Autodesk Inventor part; units mm, degrees
(part 4 of 5)
  arc A370 (116.0375, 307.325) -> (116.5375, 307.825) centre (116.0375, 307.825) ccw
  arc A371 (116.5375, 320.825) -> (116.0375, 321.325) centre (116.0375, 320.825) ccw
  line L372 (102.5375, 326.875) -> (102.5375, 339.875)
  line L373 (116.5375, 326.875) -> (116.5375, 339.875)
  line L374 (103.0375, 326.375) -> (116.0375, 326.375)
  line L375 (103.0375, 340.375) -> (116.0375, 340.375)
  arc A372 (102.5375, 326.875) -> (103.0375, 326.375) centre (103.0375, 326.875) ccw
  arc A373 (103.0375, 340.375) -> (102.5375, 339.875) centre (103.0375, 339.875) ccw
  arc A374 (116.0375, 326.375) -> (116.5375, 326.875) centre (116.0375, 326.875) ccw
  arc A375 (116.5375, 339.875) -> (116.0375, 340.375) centre (116.0375, 339.875) ccw
  line L376 (119.0625, -4.7625) -> (119.0625, 342.9)
  line L377 (0, -4.7625) -> (0, 342.9)
  line L378 (119.0625, -4.7625) -> (0, -4.7625)
  line L379 (119.0625, 342.9) -> (0, 342.9)
  point P0 (60.5977, 160.7988)
sketch "Sketch1" plane through (0, 0, 0) normal (0, 1, 0) x (-1, 0, 0)
  line L0 (0, 0) -> (144.19, 0)
  line L1 (144.19, 0) -> (144.19, -379.14)
  line L2 (144.19, -379.14) -> (0, -379.14)
  line L3 (0, -379.14) -> (0, 0)
  dimension "d0" = 144.19
  dimension "d1" = 379.14
  constraints: 8 end point, 2 parallel, 1 horizontal, 1 perpendicular
  measures "d0" distance of L1.end L2.end
  measures "d1" distance of L0.end L1.end
extrude "Extrusion1" add sketch "Sketch1" along normal blind 2
sketch "Sketch5" plane through (0, 2, 0) normal (0, 1, 0) x (1, 0, 0)
  line L0 (-144.19, 379.14) -> (-144.19, 0) projected
  line L1 (0, 379.14) -> (-144.19, 379.14) projected
  line L2 (0, 0) -> (0, 379.14) projected
  line L3 (-144.19, 0) -> (0, 0) projected
  line L4 (-128.9335, 19.693) -> (-128.9335, 32.693)
  line L5 (-114.9335, 19.693) -> (-114.9335, 32.693)
  line L6 (-128.4335, 19.193) -> (-115.4335, 19.193)
  line L7 (-128.4335, 33.193) -> (-115.4335, 33.193)
  arc A0 (-128.9335, 19.693) -> (-128.4335, 19.193) centre (-128.4335, 19.693) ccw
  arc A1 (-128.4335, 33.193) -> (-128.9335, 32.693) centre (-128.4335, 32.693) ccw
  arc A2 (-115.4335, 19.193) -> (-114.9335, 19.693) centre (-115.4335, 19.693) ccw
  arc A3 (-114.9335, 32.693) -> (-115.4335, 33.193) centre (-115.4335, 32.693) ccw
  line L8 (-128.9335, 57.793) -> (-128.9335, 70.793)
  line L9 (-114.9335, 57.793) -> (-114.9335, 70.793)
  line L10 (-128.4335, 57.293) -> (-115.4335, 57.293)
  line L11 (-128.4335, 71.293) -> (-115.4335, 71.293)
  arc A4 (-128.9335, 57.793) -> (-128.4335, 57.293) centre (-128.4335, 57.793) ccw
  arc A5 (-128.4335, 71.293) -> (-128.9335, 70.793) centre (-128.4335, 70.793) ccw
  arc A6 (-115.4335, 57.293) -> (-114.9335, 57.793) centre (-115.4335, 57.793) ccw
  arc A7 (-114.9335, 70.793) -> (-115.4335, 71.293) centre (-115.4335, 70.793) ccw
  line L12 (-128.9335, 76.843) -> (-128.9335, 89.843)
  line L13 (-114.9335, 76.843) -> (-114.9335, 89.843)
  line L14 (-128.4335, 76.343) -> (-115.4335, 76.343)
  line L15 (-128.4335, 90.343) -> (-115.4335, 90.343)
  arc A8 (-128.9335, 76.843) -> (-128.4335, 76.343) centre (-128.4335, 76.843) ccw
  arc A9 (-128.4335, 90.343) -> (-128.9335, 89.843) centre (-128.4335, 89.843) ccw
  arc A10 (-115.4335, 76.343) -> (-114.9335, 76.843) centre (-115.4335, 76.843) ccw
  arc A11 (-114.9335, 89.843) -> (-115.4335, 90.343) centre (-115.4335, 89.843) ccw
  line L16 (-128.9335, 95.893) -> (-128.9335, 108.893)
  line L17 (-114.9335, 95.893) -> (-114.9335, 108.893)
  line L18 (-128.4335, 95.393) -> (-115.4335, 95.393)
  line L19 (-128.4335, 109.393) -> (-115.4335, 109.393)
  arc A12 (-128.9335, 95.893) -> (-128.4335, 95.393) centre (-128.4335, 95.893) ccw
  arc A13 (-128.4335, 109.393) -> (-128.9335, 108.893) centre (-128.4335, 108.893) ccw
  arc A14 (-115.4335, 95.393) -> (-114.9335, 95.893) centre (-115.4335, 95.893) ccw
  arc A15 (-114.9335, 108.893) -> (-115.4335, 109.393) centre (-115.4335, 108.893) ccw
  line L20 (-128.9335, 114.943) -> (-128.9335, 127.943)
  line L21 (-114.9335, 114.943) -> (-114.9335, 127.943)
  line L22 (-128.4335, 114.443) -> (-115.4335, 114.443)
  line L23 (-128.4335, 128.443) -> (-115.4335, 128.443)
  arc A16 (-128.9335, 114.943) -> (-128.4335, 114.443) centre (-128.4335, 114.943) ccw
  arc A17 (-128.4335, 128.443) -> (-128.9335, 127.943) centre (-128.4335, 127.943) ccw
  arc A18 (-115.4335, 114.443) -> (-114.9335, 114.943) centre (-115.4335, 114.943) ccw
  arc A19 (-114.9335, 127.943) -> (-115.4335, 128.443) centre (-115.4335, 127.943) ccw
  line L24 (-128.9335, 143.518) -> (-128.9335, 156.518)
  line L25 (-114.9335, 143.518) -> (-114.9335, 156.518)
  line L26 (-128.4335, 143.018) -> (-115.4335, 143.018)
  line L27 (-128.4335, 157.018) -> (-115.4335, 157.018)
  arc A20 (-128.9335, 143.518) -> (-128.4335, 143.018) centre (-128.4335, 143.518) ccw
  arc A21 (-128.4335, 157.018) -> (-128.9335, 156.518) centre (-128.4335, 156.518) ccw
  arc A22 (-115.4335, 143.018) -> (-114.9335, 143.518) centre (-115.4335, 143.518) ccw
  arc A23 (-114.9335, 156.518) -> (-115.4335, 157.018) centre (-115.4335, 156.518) ccw
  line L28 (-128.9335, 162.568) -> (-128.9335, 175.568)
  line L29 (-114.9335, 162.568) -> (-114.9335, 175.568)
  line L30 (-128.4335, 162.068) -> (-115.4335, 162.068)
  line L31 (-128.4335, 176.068) -> (-115.4335, 176.068)
  arc A24 (-128.9335, 162.568) -> (-128.4335, 162.068) centre (-128.4335, 162.568) ccw
  arc A25 (-128.4335, 176.068) -> (-128.9335, 175.568) centre (-128.4335, 175.568) ccw
  arc A26 (-115.4335, 162.068) -> (-114.9335, 162.568) centre (-115.4335, 162.568) ccw
  arc A27 (-114.9335, 175.568) -> (-115.4335, 176.068) centre (-115.4335, 175.568) ccw
  line L32 (-128.9335, 181.618) -> (-128.9335, 194.618)
  line L33 (-114.9335, 181.618) -> (-114.9335, 194.618)
  line L34 (-128.4335, 181.118) -> (-115.4335, 181.118)
  line L35 (-128.4335, 195.118) -> (-115.4335, 195.118)
  arc A28 (-128.9335, 181.618) -> (-128.4335, 181.118) centre (-128.4335, 181.618) ccw
  arc A29 (-128.4335, 195.118) -> (-128.9335, 194.618) centre (-128.4335, 194.618) ccw
  arc A30 (-115.4335, 181.118) -> (-114.9335, 181.618) centre (-115.4335, 181.618) ccw
  arc A31 (-114.9335, 194.618) -> (-115.4335, 195.118) centre (-115.4335, 194.618) ccw
  line L36 (-128.9335, 200.668) -> (-128.9335, 213.668)
  line L37 (-114.9335, 200.668) -> (-114.9335, 213.668)
  line L38 (-128.4335, 200.168) -> (-115.4335, 200.168)
  line L39 (-128.4335, 214.168) -> (-115.4335, 214.168)
  arc A32 (-128.9335, 200.668) -> (-128.4335, 200.168) centre (-128.4335, 200.668) ccw
  arc A33 (-128.4335, 214.168) -> (-128.9335, 213.668) centre (-128.4335, 213.668) ccw
  arc A34 (-115.4335, 200.168) -> (-114.9335, 200.668) centre (-115.4335, 200.668) ccw
  arc A35 (-114.9335, 213.668) -> (-115.4335, 214.168) centre (-115.4335, 213.668) ccw
  line L40 (-128.9335, 229.243) -> (-128.9335, 242.243)
  line L41 (-114.9335, 229.243) -> (-114.9335, 242.243)
  line L42 (-128.4335, 228.743) -> (-115.4335, 228.743)
  line L43 (-128.4335, 242.743) -> (-115.4335, 242.743)
  arc A36 (-128.9335, 229.243) -> (-128.4335, 228.743) centre (-128.4335, 229.243) ccw
  arc A37 (-128.4335, 242.743) -> (-128.9335, 242.243) centre (-128.4335, 242.243) ccw
  arc A38 (-115.4335, 228.743) -> (-114.9335, 229.243) centre (-115.4335, 229.243) ccw
  arc A39 (-114.9335, 242.243) -> (-115.4335, 242.743) centre (-115.4335, 242.243) ccw
  line L44 (-128.9335, 248.293) -> (-128.9335, 261.293)
  line L45 (-114.9335, 248.293) -> (-114.9335, 261.293)
  line L46 (-128.4335, 247.793) -> (-115.4335, 247.793)
  line L47 (-128.4335, 261.793) -> (-115.4335, 261.793)
  arc A40 (-128.9335, 248.293) -> (-128.4335, 247.793) centre (-128.4335, 248.293) ccw
  arc A41 (-128.4335, 261.793) -> (-128.9335, 261.293) centre (-128.4335, 261.293) ccw
  arc A42 (-115.4335, 247.793) -> (-114.9335, 248.293) centre (-115.4335, 248.293) ccw
  arc A43 (-114.9335, 261.293) -> (-115.4335, 261.793) centre (-115.4335, 261.293) ccw
  line L48 (-128.9335, 267.343) -> (-128.9335, 280.343)
  line L49 (-114.9335, 267.343) -> (-114.9335, 280.343)
  line L50 (-128.4335, 266.843) -> (-115.4335, 266.843)
  line L51 (-128.4335, 280.843) -> (-115.4335, 280.843)
  arc A44 (-128.9335, 267.343) -> (-128.4335, 266.843) centre (-128.4335, 267.343) ccw
  arc A45 (-128.4335, 280.843) -> (-128.9335, 280.343) centre (-128.4335, 280.343) ccw
  arc A46 (-115.4335, 266.843) -> (-114.9335, 267.343) centre (-115.4335, 267.343) ccw
  arc A47 (-114.9335, 280.343) -> (-115.4335, 280.843) centre (-115.4335, 280.343) ccw
  line L52 (-128.9335, 286.393) -> (-128.9335, 299.393)
  line L53 (-114.9335, 286.393) -> (-114.9335, 299.393)
  line L54 (-128.4335, 285.893) -> (-115.4335, 285.893)
  line L55 (-128.4335, 299.893) -> (-115.4335, 299.893)
  arc A48 (-128.9335, 286.393) -> (-128.4335, 285.893) centre (-128.4335, 286.393) ccw
  arc A49 (-128.4335, 299.893) -> (-128.9335, 299.393) centre (-128.4335, 299.393) ccw
  arc A50 (-115.4335, 285.893) -> (-114.9335, 286.393) centre (-115.4335, 286.393) ccw
  arc A51 (-114.9335, 299.393) -> (-115.4335, 299.893) centre (-115.4335, 299.393) ccw
  line L56 (-105.121, 19.693) -> (-105.121, 32.693)
  line L57 (-91.121, 19.693) -> (-91.121, 32.693)
  line L58 (-104.621, 19.193) -> (-91.621, 19.193)
  line L59 (-104.621, 33.193) -> (-91.621, 33.193)
  arc A52 (-105.121, 19.693) -> (-104.621, 19.193) centre (-104.621, 19.693) ccw
  arc A53 (-104.621, 33.193) -> (-105.121, 32.693) centre (-104.621, 32.693) ccw
  arc A54 (-91.621, 19.193) -> (-91.121, 19.693) centre (-91.621, 19.693) ccw
  arc A55 (-91.121, 32.693) -> (-91.621, 33.193) centre (-91.621, 32.693) ccw
  line L60 (-105.121, 38.743) -> (-105.121, 51.743)
  line L61 (-91.121, 38.743) -> (-91.121, 51.743)
  line L62 (-104.621, 38.243) -> (-91.621, 38.243)
  line L63 (-104.621, 52.243) -> (-91.621, 52.243)
  arc A56 (-105.121, 38.743) -> (-104.621, 38.243) centre (-104.621, 38.743) ccw
  arc A57 (-104.621, 52.243) -> (-105.121, 51.743) centre (-104.621, 51.743) ccw
  arc A58 (-91.621, 38.243) -> (-91.121, 38.743) centre (-91.621, 38.743) ccw
  arc A59 (-91.121, 51.743) -> (-91.621, 52.243) centre (-91.621, 51.743) ccw
  line L64 (-105.121, 57.793) -> (-105.121, 70.793)
  line L65 (-91.121, 57.793) -> (-91.121, 70.793)
  line L66 (-104.621, 57.293) -> (-91.621, 57.293)
  line L67 (-104.621, 71.293) -> (-91.621, 71.293)
  arc A60 (-105.121, 57.793) -> (-104.621, 57.293) centre (-104.621, 57.793) ccw
  arc A61 (-104.621, 71.293) -> (-105.121, 70.793) centre (-104.621, 70.793) ccw
  arc A62 (-91.621, 57.293) -> (-91.121, 57.793) centre (-91.621, 57.793) ccw
  arc A63 (-91.121, 70.793) -> (-91.621, 71.293) centre (-91.621, 70.793) ccw
  line L68 (-105.121, 76.843) -> (-105.121, 89.843)
  line L69 (-91.121, 76.843) -> (-91.121, 89.843)
  line L70 (-104.621, 76.343) -> (-91.621, 76.343)
  line L71 (-104.621, 90.343) -> (-91.621, 90.343)
  arc A64 (-105.121, 76.843) -> (-104.621, 76.343) centre (-104.621, 76.843) ccw
  arc A65 (-104.621, 90.343) -> (-105.121, 89.843) centre (-104.621, 89.843) ccw
  arc A66 (-91.621, 76.343) -> (-91.121, 76.843) centre (-91.621, 76.843) ccw
  arc A67 (-91.121, 89.843) -> (-91.621, 90.343) centre (-91.621, 89.843) ccw
  line L72 (-105.121, 95.893) -> (-105.121, 108.893)
  line L73 (-91.121, 95.893) -> (-91.121, 108.893)
  line L74 (-104.621, 95.393) -> (-91.621, 95.393)
  line L75 (-104.621, 109.393) -> (-91.621, 109.393)
  arc A68 (-105.121, 95.893) -> (-104.621, 95.393) centre (-104.621, 95.893) ccw
  arc A69 (-104.621, 109.393) -> (-105.121, 108.893) centre (-104.621, 108.893) ccw
  arc A70 (-91.621, 95.393) -> (-91.121, 95.893) centre (-91.621, 95.893) ccw
  arc A71 (-91.121, 108.893) -> (-91.621, 109.393) centre (-91.621, 108.893) ccw
  line L76 (-105.121, 114.943) -> (-105.121, 127.943)
  line L77 (-91.121, 114.943) -> (-91.121, 127.943)
  line L78 (-104.621, 114.443) -> (-91.621, 114.443)
  line L79 (-104.621, 128.443) -> (-91.621, 128.443)
  arc A72 (-105.121, 114.943) -> (-104.621, 114.443) centre (-104.621, 114.943) ccw
  arc A73 (-104.621, 128.443) -> (-105.121, 127.943) centre (-104.621, 127.943) ccw
  arc A74 (-91.621, 114.443) -> (-91.121, 114.943) centre (-91.621, 114.943) ccw
  arc A75 (-91.121, 127.943) -> (-91.621, 128.443) centre (-91.621, 127.943) ccw
  line L80 (-105.121, 133.993) -> (-105.121, 146.993)
  line L81 (-91.121, 133.993) -> (-91.121, 146.993)
  line L82 (-104.621, 133.493) -> (-91.621, 133.493)
  line L83 (-104.621, 147.493) -> (-91.621, 147.493)
  arc A76 (-105.121, 133.993) -> (-104.621, 133.493) centre (-104.621, 133.993) ccw
  arc A77 (-104.621, 147.493) -> (-105.121, 146.993) centre (-104.621, 146.993) ccw
  arc A78 (-91.621, 133.493) -> (-91.121, 133.993) centre (-91.621, 133.993) ccw
  arc A79 (-91.121, 146.993) -> (-91.621, 147.493) centre (-91.621, 146.993) ccw
  line L84 (-105.121, 153.043) -> (-105.121, 166.043)
  line L85 (-91.121, 153.043) -> (-91.121, 166.043)
  line L86 (-104.621, 152.543) -> (-91.621, 152.543)
  line L87 (-104.621, 166.543) -> (-91.621, 166.543)
  arc A80 (-105.121, 153.043) -> (-104.621, 152.543) centre (-104.621, 153.043) ccw
  arc A81 (-104.621, 166.543) -> (-105.121, 166.043) centre (-104.621, 166.043) ccw
  arc A82 (-91.621, 152.543) -> (-91.121, 153.043) centre (-91.621, 153.043) ccw
  arc A83 (-91.121, 166.043) -> (-91.621, 166.543) centre (-91.621, 166.043) ccw
  line L88 (-105.121, 172.093) -> (-105.121, 185.093)
  line L89 (-91.121, 172.093) -> (-91.121, 185.093)
  line L90 (-104.621, 171.593) -> (-91.621, 171.593)
  line L91 (-104.621, 185.593) -> (-91.621, 185.593)
  arc A84 (-105.121, 172.093) -> (-104.621, 171.593) centre (-104.621, 172.093) ccw
  arc A85 (-104.621, 185.593) -> (-105.121, 185.093) centre (-104.621, 185.093) ccw
  arc A86 (-91.621, 171.593) -> (-91.121, 172.093) centre (-91.621, 172.093) ccw
  arc A87 (-91.121, 185.093) -> (-91.621, 185.593) centre (-91.621, 185.093) ccw
  line L92 (-105.121, 191.143) -> (-105.121, 204.143)
  line L93 (-91.121, 191.143) -> (-91.121, 204.143)
  line L94 (-104.621, 190.643) -> (-91.621, 190.643)
  line L95 (-104.621, 204.643) -> (-91.621, 204.643)
  arc A88 (-105.121, 191.143) -> (-104.621, 190.643) centre (-104.621, 191.143) ccw
  arc A89 (-104.621, 204.643) -> (-105.121, 204.143) centre (-104.621, 204.143) ccw
  arc A90 (-91.621, 190.643) -> (-91.121, 191.143) centre (-91.621, 191.143) ccw
  arc A91 (-91.121, 204.143) -> (-91.621, 204.643) centre (-91.621, 204.143) ccw
  line L96 (-105.121, 210.193) -> (-105.121, 223.193)
  line L97 (-91.121, 210.193) -> (-91.121, 223.193)
  line L98 (-104.621, 209.693) -> (-91.621, 209.693)
  line L99 (-104.621, 223.693) -> (-91.621, 223.693)
  arc A92 (-105.121, 210.193) -> (-104.621, 209.693) centre (-104.621, 210.193) ccw
  arc A93 (-104.621, 223.693) -> (-105.121, 223.193) centre (-104.621, 223.193) ccw
  arc A94 (-91.621, 209.693) -> (-91.121, 210.193) centre (-91.621, 210.193) ccw
  arc A95 (-91.121, 223.193) -> (-91.621, 223.693) centre (-91.621, 223.193) ccw
  line L100 (-105.121, 229.243) -> (-105.121, 242.243)
  line L101 (-91.121, 229.243) -> (-91.121, 242.243)
  line L102 (-104.621, 228.743) -> (-91.621, 228.743)
  line L103 (-104.621, 242.743) -> (-91.621, 242.743)
  arc A96 (-105.121, 229.243) -> (-104.621, 228.743) centre (-104.621, 229.243) ccw
  arc A97 (-104.621, 242.743) -> (-105.121, 242.243) centre (-104.621, 242.243) ccw
  arc A98 (-91.621, 228.743) -> (-91.121, 229.243) centre (-91.621, 229.243) ccw
  arc A99 (-91.121, 242.243) -> (-91.621, 242.743) centre (-91.621, 242.243) ccw
  line L104 (-105.121, 248.293) -> (-105.121, 261.293)
  line L105 (-91.121, 248.293) -> (-91.121, 261.293)
  line L106 (-104.621, 247.793) -> (-91.621, 247.793)
  line L107 (-104.621, 261.793) -> (-91.621, 261.793)
  arc A100 (-105.121, 248.293) -> (-104.621, 247.793) centre (-104.621, 248.293) ccw
  arc A101 (-104.621, 261.793) -> (-105.121, 261.293) centre (-104.621, 261.293) ccw
  arc A102 (-91.621, 247.793) -> (-91.121, 248.293) centre (-91.621, 248.293) ccw
  arc A103 (-91.121, 261.293) -> (-91.621, 261.793) centre (-91.621, 261.293) ccw
  line L108 (-105.121, 276.868) -> (-105.121, 289.868)
  line L109 (-91.121, 276.868) -> (-91.121, 289.868)
  line L110 (-104.621, 276.368) -> (-91.621, 276.368)
  line L111 (-104.621, 290.368) -> (-91.621, 290.368)
  arc A104 (-105.121, 276.868) -> (-104.621, 276.368) centre (-104.621, 276.868) ccw
  arc A105 (-104.621, 290.368) -> (-105.121, 289.868) centre (-104.621, 289.868) ccw
  arc A106 (-91.621, 276.368) -> (-91.121, 276.868) centre (-91.621, 276.868) ccw
  arc A107 (-91.121, 289.868) -> (-91.621, 290.368) centre (-91.621, 289.868) ccw
  line L112 (-104.121, 268.43) -> (-104.121, 274.43)
  line L113 (-89.121, 268.43) -> (-89.121, 274.43)
  line L114 (-103.621, 267.93) -> (-89.621, 267.93)
  line L115 (-103.621, 274.93) -> (-89.621, 274.93)
  arc A108 (-104.121, 268.43) -> (-103.621, 267.93) centre (-103.621, 268.43) ccw
  arc A109 (-103.621, 274.93) -> (-104.121, 274.43) centre (-103.621, 274.43) ccw
  arc A110 (-89.621, 267.93) -> (-89.121, 268.43) centre (-89.621, 268.43) ccw
  arc A111 (-89.121, 274.43) -> (-89.621, 274.93) centre (-89.621, 274.43) ccw
  line L116 (-104.121, 292.306) -> (-104.121, 298.306)
  line L117 (-89.121, 292.306) -> (-89.121, 298.306)
  line L118 (-103.621, 291.806) -> (-89.621, 291.806)
  line L119 (-103.621, 298.806) -> (-89.621, 298.806)
  arc A112 (-104.121, 292.306) -> (-103.621, 291.806) centre (-103.621, 292.306) ccw
  arc A113 (-103.621, 298.806) -> (-104.121, 298.306) centre (-103.621, 298.306) ccw
  arc A114 (-89.621, 291.806) -> (-89.121, 292.306) centre (-89.621, 292.306) ccw
  arc A115 (-89.121, 298.306) -> (-89.621, 298.806) centre (-89.621, 298.306) ccw
  line L120 (-105.121, 310.2055) -> (-105.121, 323.2055)
  line L121 (-91.121, 310.2055) -> (-91.121, 323.2055)
  line L122 (-104.621, 309.7055) -> (-91.621, 309.7055)
  line L123 (-104.621, 323.7055) -> (-91.621, 323.7055)
  arc A116 (-105.121, 310.2055) -> (-104.621, 309.7055) centre (-104.621, 310.2055) ccw
  arc A117 (-104.621, 323.7055) -> (-105.121, 323.2055) centre (-104.621, 323.2055) ccw
  arc A118 (-91.621, 309.7055) -> (-91.121, 310.2055) centre (-91.621, 310.2055) ccw
  arc A119 (-91.121, 323.2055) -> (-91.621, 323.7055) centre (-91.621, 323.2055) ccw
  line L124 (-105.121, 329.2555) -> (-105.121, 342.2555)
  line L125 (-91.121, 329.2555) -> (-91.121, 342.2555)
  line L126 (-104.621, 328.7555) -> (-91.621, 328.7555)
  line L127 (-104.621, 342.7555) -> (-91.621, 342.7555)
  arc A120 (-105.121, 329.2555) -> (-104.621, 328.7555) centre (-104.621, 329.2555) ccw
  arc A121 (-104.621, 342.7555) -> (-105.121, 342.2555) centre (-104.621, 342.2555) ccw
  arc A122 (-91.621, 328.7555) -> (-91.121, 329.2555) centre (-91.621, 329.2555) ccw
  arc A123 (-91.121, 342.2555) -> (-91.621, 342.7555) centre (-91.621, 342.2555) ccw
  line L128 (-105.121, 348.3055) -> (-105.121, 361.3055)
  line L129 (-91.121, 348.3055) -> (-91.121, 361.3055)
  line L130 (-104.621, 347.8055) -> (-91.621, 347.8055)
  line L131 (-104.621, 361.8055) -> (-91.621, 361.8055)
  arc A124 (-105.121, 348.3055) -> (-104.621, 347.8055) centre (-104.621, 348.3055) ccw
  arc A125 (-104.621, 361.8055) -> (-105.121, 361.3055) centre (-104.621, 361.3055) ccw
  arc A126 (-91.621, 347.8055) -> (-91.121, 348.3055) centre (-91.621, 348.3055) ccw
  arc A127 (-91.121, 361.3055) -> (-91.621, 361.8055) centre (-91.621, 361.3055) ccw
  line L132 (-86.071, 24.4555) -> (-86.071, 37.4555)
  line L133 (-72.071, 24.4555) -> (-72.071, 37.4555)
  line L134 (-85.571, 23.9555) -> (-72.571, 23.9555)
  line L135 (-85.571, 37.9555) -> (-72.571, 37.9555)
  arc A128 (-86.071, 24.4555) -> (-85.571, 23.9555) centre (-85.571, 24.4555) ccw
  arc A129 (-85.571, 37.9555) -> (-86.071, 37.4555) centre (-85.571, 37.4555) ccw
  arc A130 (-72.571, 23.9555) -> (-72.071, 24.4555) centre (-72.571, 24.4555) ccw
  arc A131 (-72.071, 37.4555) -> (-72.571, 37.9555) centre (-72.571, 37.4555) ccw
  line L136 (-86.071, 48.268) -> (-86.071, 61.268)
  line L137 (-72.071, 48.268) -> (-72.071, 61.268)
  line L138 (-85.571, 47.768) -> (-72.571, 47.768)
  line L139 (-85.571, 61.768) -> (-72.571, 61.768)
  arc A132 (-86.071, 48.268) -> (-85.571, 47.768) centre (-85.571, 48.268) ccw
  arc A133 (-85.571, 61.768) -> (-86.071, 61.268) centre (-85.571, 61.268) ccw
  arc A134 (-72.571, 47.768) -> (-72.071, 48.268) centre (-72.571, 48.268) ccw
  arc A135 (-72.071, 61.268) -> (-72.571, 61.768) centre (-72.571, 61.268) ccw
  line L140 (-86.071, 67.318) -> (-86.071, 80.318)
  line L141 (-72.071, 67.318) -> (-72.071, 80.318)
  line L142 (-85.571, 66.818) -> (-72.571, 66.818)
  line L143 (-85.571, 80.818) -> (-72.571, 80.818)
  arc A136 (-86.071, 67.318) -> (-85.571, 66.818) centre (-85.571, 67.318) ccw
  arc A137 (-85.571, 80.818) -> (-86.071, 80.318) centre (-85.571, 80.318) ccw
  arc A138 (-72.571, 66.818) -> (-72.071, 67.318) centre (-72.571, 67.318) ccw
  arc A139 (-72.071, 80.318) -> (-72.571, 80.818) centre (-72.571, 80.318) ccw
  line L144 (-86.071, 86.368) -> (-86.071, 99.368)
  line L145 (-72.071, 86.368) -> (-72.071, 99.368)
  line L146 (-85.571, 85.868) -> (-72.571, 85.868)
  line L147 (-85.571, 99.868) -> (-72.571, 99.868)
  arc A140 (-86.071, 86.368) -> (-85.571, 85.868) centre (-85.571, 86.368) ccw
  arc A141 (-85.571, 99.868) -> (-86.071, 99.368) centre (-85.571, 99.368) ccw
  arc A142 (-72.571, 85.868) -> (-72.071, 86.368) centre (-72.571, 86.368) ccw
  arc A143 (-72.071, 99.368) -> (-72.571, 99.868) centre (-72.571, 99.368) ccw
  line L148 (-86.071, 105.418) -> (-86.071, 118.418)
  line L149 (-72.071, 105.418) -> (-72.071, 118.418)
  line L150 (-85.571, 104.918) -> (-72.571, 104.918)
  line L151 (-85.571, 118.918) -> (-72.571, 118.918)
  arc A144 (-86.071, 105.418) -> (-85.571, 104.918) centre (-85.571, 105.418) ccw
  arc A145 (-85.571, 118.918) -> (-86.071, 118.418) centre (-85.571, 118.418) ccw
  arc A146 (-72.571, 104.918) -> (-72.071, 105.418) centre (-72.571, 105.418) ccw
  arc A147 (-72.071, 118.418) -> (-72.571, 118.918) centre (-72.571, 118.418) ccw
  line L152 (-86.071, 124.468) -> (-86.071, 137.468)
  line L153 (-72.071, 124.468) -> (-72.071, 137.468)
  line L154 (-85.571, 123.968) -> (-72.571, 123.968)
  line L155 (-85.571, 137.968) -> (-72.571, 137.968)
  arc A148 (-86.071, 124.468) -> (-85.571, 123.968) centre (-85.571, 124.468) ccw
  arc A149 (-85.571, 137.968) -> (-86.071, 137.468) centre (-85.571, 137.468) ccw
  arc A150 (-72.571, 123.968) -> (-72.071, 124.468) centre (-72.571, 124.468) ccw
  arc A151 (-72.071, 137.468) -> (-72.571, 137.968) centre (-72.571, 137.468) ccw
  line L156 (-86.071, 143.518) -> (-86.071, 156.518)
  line L157 (-72.071, 143.518) -> (-72.071, 156.518)
  line L158 (-85.571, 143.018) -> (-72.571, 143.018)
  line L159 (-85.571, 157.018) -> (-72.571, 157.018)
  arc A152 (-86.071, 143.518) -> (-85.571, 143.018) centre (-85.571, 143.518) ccw
  arc A153 (-85.571, 157.018) -> (-86.071, 156.518) centre (-85.571, 156.518) ccw
  arc A154 (-72.571, 143.018) -> (-72.071, 143.518) centre (-72.571, 143.518) ccw
  arc A155 (-72.071, 156.518) -> (-72.571, 157.018) centre (-72.571, 156.518) ccw
  line L160 (-86.071, 162.568) -> (-86.071, 175.568)
  line L161 (-72.071, 162.568) -> (-72.071, 175.568)
  line L162 (-85.571, 162.068) -> (-72.571, 162.068)
  line L163 (-85.571, 176.068) -> (-72.571, 176.068)
  arc A156 (-86.071, 162.568) -> (-85.571, 162.068) centre (-85.571, 162.568) ccw
  arc A157 (-85.571, 176.068) -> (-86.071, 175.568) centre (-85.571, 175.568) ccw
  arc A158 (-72.571, 162.068) -> (-72.071, 162.568) centre (-72.571, 162.568) ccw
  arc A159 (-72.071, 175.568) -> (-72.571, 176.068) centre (-72.571, 175.568) ccw
  line L164 (-86.071, 181.618) -> (-86.071, 194.618)
  line L165 (-72.071, 181.618) -> (-72.071, 194.618)
  line L166 (-85.571, 181.118) -> (-72.571, 181.118)
  line L167 (-85.571, 195.118) -> (-72.571, 195.118)
  arc A160 (-86.071, 181.618) -> (-85.571, 181.118) centre (-85.571, 181.618) ccw
  arc A161 (-85.571, 195.118) -> (-86.071, 194.618) centre (-85.571, 194.618) ccw
  arc A162 (-72.571, 181.118) -> (-72.071, 181.618) centre (-72.571, 181.618) ccw
  arc A163 (-72.071, 194.618) -> (-72.571, 195.118) centre (-72.571, 194.618) ccw
  line L168 (-86.071, 200.668) -> (-86.071, 213.668)
  line L169 (-72.071, 200.668) -> (-72.071, 213.668)
  line L170 (-85.571, 200.168) -> (-72.571, 200.168)
  line L171 (-85.571, 214.168) -> (-72.571, 214.168)
  arc A164 (-86.071, 200.668) -> (-85.571, 200.168) centre (-85.571, 200.668) ccw
  arc A165 (-85.571, 214.168) -> (-86.071, 213.668) centre (-85.571, 213.668) ccw
  arc A166 (-72.571, 200.168) -> (-72.071, 200.668) centre (-72.571, 200.668) ccw
  arc A167 (-72.071, 213.668) -> (-72.571, 214.168) centre (-72.571, 213.668) ccw
  line L172 (-86.071, 219.718) -> (-86.071, 232.718)
  line L173 (-72.071, 219.718) -> (-72.071, 232.718)
  line L174 (-85.571, 219.218) -> (-72.571, 219.218)
  line L175 (-85.571, 233.218) -> (-72.571, 233.218)
  arc A168 (-86.071, 219.718) -> (-85.571, 219.218) centre (-85.571, 219.718) ccw
  arc A169 (-85.571, 233.218) -> (-86.071, 232.718) centre (-85.571, 232.718) ccw
  arc A170 (-72.571, 219.218) -> (-72.071, 219.718) centre (-72.571, 219.718) ccw
  arc A171 (-72.071, 232.718) -> (-72.571, 233.218) centre (-72.571, 232.718) ccw
  line L176 (-86.071, 238.768) -> (-86.071, 251.768)
  line L177 (-72.071, 238.768) -> (-72.071, 251.768)
  line L178 (-85.571, 238.268) -> (-72.571, 238.268)
  line L179 (-85.571, 252.268) -> (-72.571, 252.268)
  arc A172 (-86.071, 238.768) -> (-85.571, 238.268) centre (-85.571, 238.768) ccw
  arc A173 (-85.571, 252.268) -> (-86.071, 251.768) centre (-85.571, 251.768) ccw
  arc A174 (-72.571, 238.268) -> (-72.071, 238.768) centre (-72.571, 238.768) ccw
  arc A175 (-72.071, 251.768) -> (-72.571, 252.268) centre (-72.571, 251.768) ccw
  line L180 (-86.071, 257.818) -> (-86.071, 270.818)
  line L181 (-72.071, 257.818) -> (-72.071, 270.818)
  line L182 (-85.571, 257.318) -> (-72.571, 257.318)
  line L183 (-85.571, 271.318) -> (-72.571, 271.318)
  arc A176 (-86.071, 257.818) -> (-85.571, 257.318) centre (-85.571, 257.818) ccw
  arc A177 (-85.571, 271.318) -> (-86.071, 270.818) centre (-85.571, 270.818) ccw
  arc A178 (-72.571, 257.318) -> (-72.071, 257.818) centre (-72.571, 257.818) ccw
  arc A179 (-72.071, 270.818) -> (-72.571, 271.318) centre (-72.571, 270.818) ccw
  line L184 (-86.071, 281.6305) -> (-86.071, 294.6305)
  line L185 (-72.071, 281.6305) -> (-72.071, 294.6305)
  line L186 (-85.571, 281.1305) -> (-72.571, 281.1305)
  line L187 (-85.571, 295.1305) -> (-72.571, 295.1305)
  arc A180 (-86.071, 281.6305) -> (-85.571, 281.1305) centre (-85.571, 281.6305) ccw
  arc A181 (-85.571, 295.1305) -> (-86.071, 294.6305) centre (-85.571, 294.6305) ccw
  arc A182 (-72.571, 281.1305) -> (-72.071, 281.6305) centre (-72.571, 281.6305) ccw
  arc A183 (-72.071, 294.6305) -> (-72.571, 295.1305) centre (-72.571, 294.6305) ccw
  line L188 (-86.071, 310.2055) -> (-86.071, 323.2055)
  line L189 (-72.071, 310.2055) -> (-72.071, 323.2055)
  line L190 (-85.571, 309.7055) -> (-72.571, 309.7055)
  line L191 (-85.571, 323.7055) -> (-72.571, 323.7055)
  arc A184 (-86.071, 310.2055) -> (-85.571, 309.7055) centre (-85.571, 310.2055) ccw
  arc A185 (-85.571, 323.7055) -> (-86.071, 323.2055) centre (-85.571, 323.2055) ccw
  arc A186 (-72.571, 309.7055) -> (-72.071, 310.2055) centre (-72.571, 310.2055) ccw
  arc A187 (-72.071, 323.2055) -> (-72.571, 323.7055) centre (-72.571, 323.2055) ccw
  line L192 (-86.071, 329.2555) -> (-86.071, 342.2555)
  line L193 (-72.071, 329.2555) -> (-72.071, 342.2555)
  line L194 (-85.571, 328.7555) -> (-72.571, 328.7555)
  line L195 (-85.571, 342.7555) -> (-72.571, 342.7555)
  arc A188 (-86.071, 329.2555) -> (-85.571, 328.7555) centre (-85.571, 329.2555) ccw
  arc A189 (-85.571, 342.7555) -> (-86.071, 342.2555) centre (-85.571, 342.2555) ccw
  arc A190 (-72.571, 328.7555) -> (-72.071, 329.2555) centre (-72.571, 329.2555) ccw
  arc A191 (-72.071, 342.2555) -> (-72.571, 342.7555) centre (-72.571, 342.2555) ccw
  line L196 (-86.071, 348.3055) -> (-86.071, 361.3055)
  line L197 (-72.071, 348.3055) -> (-72.071, 361.3055)
  line L198 (-85.571, 347.8055) -> (-72.571, 347.8055)
  line L199 (-85.571, 361.8055) -> (-72.571, 361.8055)
  arc A192 (-86.071, 348.3055) -> (-85.571, 347.8055) centre (-85.571, 348.3055) ccw
  arc A193 (-85.571, 361.8055) -> (-86.071, 361.3055) centre (-85.571, 361.3055) ccw
  arc A194 (-72.571, 347.8055) -> (-72.071, 348.3055) centre (-72.571, 348.3055) ccw
  arc A195 (-72.071, 361.3055) -> (-72.571, 361.8055) centre (-72.571, 361.3055) ccw
  line L200 (-67.021, 26.8368) -> (-67.021, 39.8368)
  line L201 (-53.021, 26.8368) -> (-53.021, 39.8368)
  line L202 (-66.521, 26.3368) -> (-53.521, 26.3368)
  line L203 (-66.521, 40.3368) -> (-53.521, 40.3368)
  arc A196 (-67.021, 26.8368) -> (-66.521, 26.3368) centre (-66.521, 26.8368) ccw
  arc A197 (-66.521, 40.3368) -> (-67.021, 39.8368) centre (-66.521, 39.8368) ccw
  arc A198 (-53.521, 26.3368) -> (-53.021, 26.8368) centre (-53.521, 26.8368) ccw
  arc A199 (-53.021, 39.8368) -> (-53.521, 40.3368) centre (-53.521, 39.8368) ccw
  line L204 (-67.021, 53.0305) -> (-67.021, 66.0305)
  line L205 (-53.021, 53.0305) -> (-53.021, 66.0305)
  line L206 (-66.521, 52.5305) -> (-53.521, 52.5305)
  line L207 (-66.521, 66.5305) -> (-53.521, 66.5305)
  arc A200 (-67.021, 53.0305) -> (-66.521, 52.5305) centre (-66.521, 53.0305) ccw
  arc A201 (-66.521, 66.5305) -> (-67.021, 66.0305) centre (-66.521, 66.0305) ccw
  arc A202 (-53.521, 52.5305) -> (-53.021, 53.0305) centre (-53.521, 53.0305) ccw
  arc A203 (-53.021, 66.0305) -> (-53.521, 66.5305) centre (-53.521, 66.0305) ccw
  line L208 (-67.021, 72.0805) -> (-67.021, 85.0805)
  line L209 (-53.021, 72.0805) -> (-53.021, 85.0805)
  line L210 (-66.521, 71.5805) -> (-53.521, 71.5805)
  line L211 (-66.521, 85.5805) -> (-53.521, 85.5805)
  arc A204 (-67.021, 72.0805) -> (-66.521, 71.5805) centre (-66.521, 72.0805) ccw
  arc A205 (-66.521, 85.5805) -> (-67.021, 85.0805) centre (-66.521, 85.0805) ccw
  arc A206 (-53.521, 71.5805) -> (-53.021, 72.0805) centre (-53.521, 72.0805) ccw
  arc A207 (-53.021, 85.0805) -> (-53.521, 85.5805) centre (-53.521, 85.0805) ccw
  line L212 (-67.021, 91.1305) -> (-67.021, 104.1305)
  line L213 (-53.021, 91.1305) -> (-53.021, 104.1305)
  line L214 (-66.521, 90.6305) -> (-53.521, 90.6305)
  line L215 (-66.521, 104.6305) -> (-53.521, 104.6305)
  arc A208 (-67.021, 91.1305) -> (-66.521, 90.6305) centre (-66.521, 91.1305) ccw
  arc A209 (-66.521, 104.6305) -> (-67.021, 104.1305) centre (-66.521, 104.1305) ccw
  arc A210 (-53.521, 90.6305) -> (-53.021, 91.1305) centre (-53.521, 91.1305) ccw
  arc A211 (-53.021, 104.1305) -> (-53.521, 104.6305) centre (-53.521, 104.1305) ccw
  line L216 (-67.021, 110.1805) -> (-67.021, 123.1805)
  line L217 (-53.021, 110.1805) -> (-53.021, 123.1805)
  line L218 (-66.521, 109.6805) -> (-53.521, 109.6805)
  line L219 (-66.521, 123.6805) -> (-53.521, 123.6805)
  arc A212 (-67.021, 110.1805) -> (-66.521, 109.6805) centre (-66.521, 110.1805) ccw
  arc A213 (-66.521, 123.6805) -> (-67.021, 123.1805) centre (-66.521, 123.1805) ccw
  arc A214 (-53.521, 109.6805) -> (-53.021, 110.1805) centre (-53.521, 110.1805) ccw
  arc A215 (-53.021, 123.1805) -> (-53.521, 123.6805) centre (-53.521, 123.1805) ccw
  line L220 (-67.021, 129.2305) -> (-67.021, 142.2305)
  line L221 (-53.021, 129.2305) -> (-53.021, 142.2305)
  line L222 (-66.521, 128.7305) -> (-53.521, 128.7305)
  line L223 (-66.521, 142.7305) -> (-53.521, 142.7305)
  arc A216 (-67.021, 129.2305) -> (-66.521, 128.7305) centre (-66.521, 129.2305) ccw
  arc A217 (-66.521, 142.7305) -> (-67.021, 142.2305) centre (-66.521, 142.2305) ccw
  arc A218 (-53.521, 128.7305) -> (-53.021, 129.2305) centre (-53.521, 129.2305) ccw
  arc A219 (-53.021, 142.2305) -> (-53.521, 142.7305) centre (-53.521, 142.2305) ccw
  line L224 (-67.021, 148.2805) -> (-67.021, 161.2805)
  line L225 (-53.021, 148.2805) -> (-53.021, 161.2805)
  line L226 (-66.521, 147.7805) -> (-53.521, 147.7805)
  line L227 (-66.521, 161.7805) -> (-53.521, 161.7805)
  arc A220 (-67.021, 148.2805) -> (-66.521, 147.7805) centre (-66.521, 148.2805) ccw
  arc A221 (-66.521, 161.7805) -> (-67.021, 161.2805) centre (-66.521, 161.2805) ccw
  arc A222 (-53.521, 147.7805) -> (-53.021, 148.2805) centre (-53.521, 148.2805) ccw
  arc A223 (-53.021, 161.2805) -> (-53.521, 161.7805) centre (-53.521, 161.2805) ccw
  line L228 (-67.021, 167.3305) -> (-67.021, 180.3305)
  line L229 (-53.021, 167.3305) -> (-53.021, 180.3305)
  line L230 (-66.521, 166.8305) -> (-53.521, 166.8305)
  line L231 (-66.521, 180.8305) -> (-53.521, 180.8305)
  arc A224 (-67.021, 167.3305) -> (-66.521, 166.8305) centre (-66.521, 167.3305) ccw
  arc A225 (-66.521, 180.8305) -> (-67.021, 180.3305) centre (-66.521, 180.3305) ccw
  arc A226 (-53.521, 166.8305) -> (-53.021, 167.3305) centre (-53.521, 167.3305) ccw
  arc A227 (-53.021, 180.3305) -> (-53.521, 180.8305) centre (-53.521, 180.3305) ccw
  line L232 (-67.021, 186.3805) -> (-67.021, 199.3805)
  line L233 (-53.021, 186.3805) -> (-53.021, 199.3805)
  line L234 (-66.521, 185.8805) -> (-53.521, 185.8805)
  line L235 (-66.521, 199.8805) -> (-53.521, 199.8805)
  arc A228 (-67.021, 186.3805) -> (-66.521, 185.8805) centre (-66.521, 186.3805) ccw
  arc A229 (-66.521, 199.8805) -> (-67.021, 199.3805) centre (-66.521, 199.3805) ccw
  arc A230 (-53.521, 185.8805) -> (-53.021, 186.3805) centre (-53.521, 186.3805) ccw
  arc A231 (-53.021, 199.3805) -> (-53.521, 199.8805) centre (-53.521, 199.3805) ccw
  line L236 (-67.021, 205.4305) -> (-67.021, 218.4305)
  line L237 (-53.021, 205.4305) -> (-53.021, 218.4305)
  line L238 (-66.521, 204.9305) -> (-53.521, 204.9305)
  line L239 (-66.521, 218.9305) -> (-53.521, 218.9305)
  arc A232 (-67.021, 205.4305) -> (-66.521, 204.9305) centre (-66.521, 205.4305) ccw
  arc A233 (-66.521, 218.9305) -> (-67.021, 218.4305) centre (-66.521, 218.4305) ccw
  arc A234 (-53.521, 204.9305) -> (-53.021, 205.4305) centre (-53.521, 205.4305) ccw
  arc A235 (-53.021, 218.4305) -> (-53.521, 218.9305) centre (-53.521, 218.4305) ccw
  line L240 (-67.021, 224.4805) -> (-67.021, 237.4805)
  line L241 (-53.021, 224.4805) -> (-53.021, 237.4805)
  line L242 (-66.521, 223.9805) -> (-53.521, 223.9805)
  line L243 (-66.521, 237.9805) -> (-53.521, 237.9805)
  arc A236 (-67.021, 224.4805) -> (-66.521, 223.9805) centre (-66.521, 224.4805) ccw
  arc A237 (-66.521, 237.9805) -> (-67.021, 237.4805) centre (-66.521, 237.4805) ccw
  arc A238 (-53.521, 223.9805) -> (-53.021, 224.4805) centre (-53.521, 224.4805) ccw
  arc A239 (-53.021, 237.4805) -> (-53.521, 237.9805) centre (-53.521, 237.4805) ccw
  line L244 (-67.021, 243.5305) -> (-67.021, 256.5305)
  line L245 (-53.021, 243.5305) -> (-53.021, 256.5305)
  line L246 (-66.521, 243.0305) -> (-53.521, 243.0305)
  line L247 (-66.521, 257.0305) -> (-53.521, 257.0305)
  arc A240 (-67.021, 243.5305) -> (-66.521, 243.0305) centre (-66.521, 243.5305) ccw
  arc A241 (-66.521, 257.0305) -> (-67.021, 256.5305) centre (-66.521, 256.5305) ccw
  arc A242 (-53.521, 243.0305) -> (-53.021, 243.5305) centre (-53.521, 243.5305) ccw
  arc A243 (-53.021, 256.5305) -> (-53.521, 257.0305) centre (-53.521, 256.5305) ccw
  line L248 (-67.021, 274.4868) -> (-67.021, 287.4868)
  line L249 (-53.021, 274.4868) -> (-53.021, 287.4868)
  line L250 (-66.521, 273.9868) -> (-53.521, 273.9868)
  line L251 (-66.521, 287.9868) -> (-53.521, 287.9868)
  arc A244 (-67.021, 274.4868) -> (-66.521, 273.9868) centre (-66.521, 274.4868) ccw
  arc A245 (-66.521, 287.9868) -> (-67.021, 287.4868) centre (-66.521, 287.4868) ccw
  arc A246 (-53.521, 273.9868) -> (-53.021, 274.4868) centre (-53.521, 274.4868) ccw
  arc A247 (-53.021, 287.4868) -> (-53.521, 287.9868) centre (-53.521, 287.4868) ccw
  line L252 (-66.021, 266.0488) -> (-66.021, 272.0488)
  line L253 (-51.021, 266.0488) -> (-51.021, 272.0488)
  line L254 (-65.521, 265.5488) -> (-51.521, 265.5487)
  line L255 (-65.521, 272.5488) -> (-51.521, 272.5488)
  arc A248 (-66.021, 266.0488) -> (-65.521, 265.5488) centre (-65.521, 266.0488) ccw
  arc A249 (-65.521, 272.5487) -> (-66.021, 272.0488) centre (-65.521, 272.0487) ccw
  arc A250 (-51.521, 265.5487) -> (-51.021, 266.0488) centre (-51.521, 266.0488) ccw
  arc A251 (-51.021, 272.0488) -> (-51.521, 272.5488) centre (-51.521, 272.0488) ccw
  line L256 (-66.021, 289.9248) -> (-66.021, 295.9248)
  line L257 (-51.021, 289.9248) -> (-51.021, 295.9248)
  line L258 (-65.521, 289.4248) -> (-51.521, 289.4248)
  line L259 (-65.521, 296.4248) -> (-51.521, 296.4248)
  arc A252 (-66.021, 289.9248) -> (-65.521, 289.4248) centre (-65.521, 289.9248) ccw
  arc A253 (-65.521, 296.4248) -> (-66.021, 295.9248) centre (-65.521, 295.9248) ccw
  arc A254 (-51.521, 289.4248) -> (-51.021, 289.9248) centre (-51.521, 289.9248) ccw
  arc A255 (-51.021, 295.9248) -> (-51.521, 296.4248) centre (-51.521, 295.9248) ccw
  line L260 (-47.971, 31.5993) -> (-47.971, 44.5993)
  line L261 (-33.971, 31.5993) -> (-33.971, 44.5992)
  line L262 (-47.471, 31.0993) -> (-34.471, 31.0993)
  line L263 (-47.471, 45.0993) -> (-34.471, 45.0993)
  arc A256 (-47.971, 31.5993) -> (-47.471, 31.0993) centre (-47.471, 31.5992) ccw
  arc A257 (-47.471, 45.0993) -> (-47.971, 44.5993) centre (-47.471, 44.5993) ccw
  arc A258 (-34.471, 31.0993) -> (-33.971, 31.5993) centre (-34.471, 31.5993) ccw
  arc A259 (-33.971, 44.5992) -> (-34.471, 45.0993) centre (-34.471, 44.5993) ccw
  line L264 (-46.971, 23.1613) -> (-46.971, 29.1613)
  line L265 (-31.971, 23.1613) -> (-31.971, 29.1612)
  line L266 (-46.471, 22.6613) -> (-32.471, 22.6613)
  line L267 (-46.471, 29.6613) -> (-32.471, 29.6613)
  arc A260 (-46.971, 23.1613) -> (-46.471, 22.6612) centre (-46.471, 23.1613) ccw
  arc A261 (-46.471, 29.6613) -> (-46.971, 29.1613) centre (-46.471, 29.1613) ccw
  arc A262 (-32.471, 22.6612) -> (-31.971, 23.1613) centre (-32.471, 23.1613) ccw
  arc A263 (-31.971, 29.1612) -> (-32.471, 29.6613) centre (-32.471, 29.1613) ccw
  line L268 (-46.971, 47.0373) -> (-46.971, 53.0373)
  line L269 (-31.971, 47.0373) -> (-31.971, 53.0373)
  line L270 (-46.471, 46.5373) -> (-32.471, 46.5373)
  line L271 (-46.471, 53.5373) -> (-32.471, 53.5373)
  arc A264 (-46.971, 47.0373) -> (-46.471, 46.5373) centre (-46.471, 47.0373) ccw
  arc A265 (-46.471, 53.5373) -> (-46.971, 53.0373) centre (-46.471, 53.0373) ccw
  arc A266 (-32.471, 46.5373) -> (-31.971, 47.0373) centre (-32.471, 47.0373) ccw
  arc A267 (-31.971, 53.0373) -> (-32.471, 53.5373) centre (-32.471, 53.0373) ccw
  line L272 (-47.971, 62.5555) -> (-47.971, 75.5555)
  line L273 (-33.971, 62.5555) -> (-33.971, 75.5555)
  line L274 (-47.471, 62.0555) -> (-34.471, 62.0555)
  line L275 (-47.471, 76.0555) -> (-34.471, 76.0555)
  arc A268 (-47.971, 62.5555) -> (-47.471, 62.0555) centre (-47.471, 62.5555) ccw
  arc A269 (-47.471, 76.0555) -> (-47.971, 75.5555) centre (-47.471, 75.5555) ccw
  arc A270 (-34.471, 62.0555) -> (-33.971, 62.5555) centre (-34.471, 62.5555) ccw
  arc A271 (-33.971, 75.5555) -> (-34.471, 76.0555) centre (-34.471, 75.5555) ccw
  line L276 (-47.971, 81.6055) -> (-47.971, 94.6055)
  line L277 (-33.971, 81.6055) -> (-33.971, 94.6055)
  line L278 (-47.471, 81.1055) -> (-34.471, 81.1055)
  line L279 (-47.471, 95.1055) -> (-34.471, 95.1055)
  arc A272 (-47.971, 81.6055) -> (-47.471, 81.1055) centre (-47.471, 81.6055) ccw
  arc A273 (-47.471, 95.1055) -> (-47.971, 94.6055) centre (-47.471, 94.6055) ccw
  arc A274 (-34.471, 81.1055) -> (-33.971, 81.6055) centre (-34.471, 81.6055) ccw
  arc A275 (-33.971, 94.6055) -> (-34.471, 95.1055) centre (-34.471, 94.6055) ccw
  line L280 (-47.971, 100.6555) -> (-47.971, 113.6555)
  line L281 (-33.971, 100.6555) -> (-33.971, 113.6555)
  line L282 (-47.471, 100.1555) -> (-34.471, 100.1555)
  line L283 (-47.471, 114.1555) -> (-34.471, 114.1555)
  arc A276 (-47.971, 100.6555) -> (-47.471, 100.1555) centre (-47.471, 100.6555) ccw
  arc A277 (-47.471, 114.1555) -> (-47.971, 113.6555) centre (-47.471, 113.6555) ccw
  arc A278 (-34.471, 100.1555) -> (-33.971, 100.6555) centre (-34.471, 100.6555) ccw
  arc A279 (-33.971, 113.6555) -> (-34.471, 114.1555) centre (-34.471, 113.6555) ccw
  line L284 (-47.971, 119.7055) -> (-47.971, 132.7055)
  line L285 (-33.971, 119.7055) -> (-33.971, 132.7055)
  line L286 (-47.471, 119.2055) -> (-34.471, 119.2055)
  line L287 (-47.471, 133.2055) -> (-34.471, 133.2055)
  arc A280 (-47.971, 119.7055) -> (-47.471, 119.2055) centre (-47.471, 119.7055) ccw
  arc A281 (-47.471, 133.2055) -> (-47.971, 132.7055) centre (-47.471, 132.7055) ccw
  arc A282 (-34.471, 119.2055) -> (-33.971, 119.7055) centre (-34.471, 119.7055) ccw
  arc A283 (-33.971, 132.7055) -> (-34.471, 133.2055) centre (-34.471, 132.7055) ccw
  line L288 (-47.971, 138.7555) -> (-47.971, 151.7555)
  line L289 (-33.971, 138.7555) -> (-33.971, 151.7555)
  line L290 (-47.471, 138.2555) -> (-34.471, 138.2555)
  line L291 (-47.471, 152.2555) -> (-34.471, 152.2555)
  arc A284 (-47.971, 138.7555) -> (-47.471, 138.2555) centre (-47.471, 138.7555) ccw
  arc A285 (-47.471, 152.2555) -> (-47.971, 151.7555) centre (-47.471, 151.7555) ccw
  arc A286 (-34.471, 138.2555) -> (-33.971, 138.7555) centre (-34.471, 138.7555) ccw
  arc A287 (-33.971, 151.7555) -> (-34.471, 152.2555) centre (-34.471, 151.7555) ccw
  line L292 (-47.971, 157.8055) -> (-47.971, 170.8055)
  line L293 (-33.971, 157.8055) -> (-33.971, 170.8055)
  line L294 (-47.471, 157.3055) -> (-34.471, 157.3055)
  line L295 (-47.471, 171.3055) -> (-34.471, 171.3055)
  arc A288 (-47.971, 157.8055) -> (-47.471, 157.3055) centre (-47.471, 157.8055) ccw
  arc A289 (-47.471, 171.3055) -> (-47.971, 170.8055) centre (-47.471, 170.8055) ccw
  arc A290 (-34.471, 157.3055) -> (-33.971, 157.8055) centre (-34.471, 157.8055) ccw
  arc A291 (-33.971, 170.8055) -> (-34.471, 171.3055) centre (-34.471, 170.8055) ccw
  line L296 (-47.971, 176.8555) -> (-47.971, 189.8555)
  line L297 (-33.971, 176.8555) -> (-33.971, 189.8555)
  line L298 (-47.471, 176.3555) -> (-34.471, 176.3555)
  line L299 (-47.471, 190.3555) -> (-34.471, 190.3555)
  arc A292 (-47.971, 176.8555) -> (-47.471, 176.3555) centre (-47.471, 176.8555) ccw
  arc A293 (-47.471, 190.3555) -> (-47.971, 189.8555) centre (-47.471, 189.8555) ccw
  arc A294 (-34.471, 176.3555) -> (-33.971, 176.8555) centre (-34.471, 176.8555) ccw
  arc A295 (-33.971, 189.8555) -> (-34.471, 190.3555) centre (-34.471, 189.8555) ccw
  line L300 (-47.971, 195.9055) -> (-47.971, 208.9055)
  line L301 (-33.971, 195.9055) -> (-33.971, 208.9055)
  line L302 (-47.471, 195.4055) -> (-34.471, 195.4055)
  line L303 (-47.471, 209.4055) -> (-34.471, 209.4055)
  arc A296 (-47.971, 195.9055) -> (-47.471, 195.4055) centre (-47.471, 195.9055) ccw
  arc A297 (-47.471, 209.4055) -> (-47.971, 208.9055) centre (-47.471, 208.9055) ccw
  arc A298 (-34.471, 195.4055) -> (-33.971, 195.9055) centre (-34.471, 195.9055) ccw
  arc A299 (-33.971, 208.9055) -> (-34.471, 209.4055) centre (-34.471, 208.9055) ccw
  line L304 (-47.971, 214.9555) -> (-47.971, 227.9555)
  line L305 (-33.971, 214.9555) -> (-33.971, 227.9555)
  line L306 (-47.471, 214.4555) -> (-34.471, 214.4555)
  line L307 (-47.471, 228.4555) -> (-34.471, 228.4555)
  arc A300 (-47.971, 214.9555) -> (-47.471, 214.4555) centre (-47.471, 214.9555) ccw
  arc A301 (-47.471, 228.4555) -> (-47.971, 227.9555) centre (-47.471, 227.9555) ccw
  arc A302 (-34.471, 214.4555) -> (-33.971, 214.9555) centre (-34.471, 214.9555) ccw
  arc A303 (-33.971, 227.9555) -> (-34.471, 228.4555) centre (-34.471, 227.9555) ccw
  line L308 (-47.971, 234.0055) -> (-47.971, 247.0055)
  line L309 (-33.971, 234.0055) -> (-33.971, 247.0055)
  line L310 (-47.471, 233.5055) -> (-34.471, 233.5055)
  line L311 (-47.471, 247.5055) -> (-34.471, 247.5055)
  arc A304 (-47.971, 234.0055) -> (-47.471, 233.5055) centre (-47.471, 234.0055) ccw
  arc A305 (-47.471, 247.5055) -> (-47.971, 247.0055) centre (-47.471, 247.0055) ccw
  arc A306 (-34.471, 233.5055) -> (-33.971, 234.0055) centre (-34.471, 234.0055) ccw
  arc A307 (-33.971, 247.0055) -> (-34.471, 247.5055) centre (-34.471, 247.0055) ccw
  line L312 (-47.971, 269.7243) -> (-47.971, 282.7243)
  line L313 (-33.971, 269.7243) -> (-33.971, 282.7243)
  line L314 (-47.471, 269.2243) -> (-34.471, 269.2243)
  line L315 (-47.471, 283.2242) -> (-34.471, 283.2243)
  arc A308 (-47.971, 269.7243) -> (-47.471, 269.2243) centre (-47.471, 269.7243) ccw
  arc A309 (-47.471, 283.2243) -> (-47.971, 282.7243) centre (-47.471, 282.7243) ccw
  arc A310 (-34.471, 269.2243) -> (-33.971, 269.7243) centre (-34.471, 269.7243) ccw
  arc A311 (-33.971, 282.7243) -> (-34.471, 283.2242) centre (-34.471, 282.7243) ccw
  line L316 (-46.971, 261.2863) -> (-46.971, 267.2863)
  line L317 (-31.971, 261.2863) -> (-31.971, 267.2863)
  line L318 (-46.471, 260.7863) -> (-32.471, 260.7863)
  line L319 (-46.471, 267.7863) -> (-32.471, 267.7862)
  arc A312 (-46.971, 261.2863) -> (-46.471, 260.7863) centre (-46.471, 261.2863) ccw
  arc A313 (-46.471, 267.7863) -> (-46.971, 267.2863) centre (-46.471, 267.2863) ccw
  arc A314 (-32.471, 260.7863) -> (-31.971, 261.2863) centre (-32.471, 261.2863) ccw
  arc A315 (-31.971, 267.2863) -> (-32.471, 267.7862) centre (-32.471, 267.2862) ccw
  line L320 (-46.971, 285.1623) -> (-46.971, 291.1623)
  line L321 (-31.971, 285.1623) -> (-31.971, 291.1623)
  line L322 (-46.471, 284.6623) -> (-32.471, 284.6623)
  line L323 (-46.471, 291.6623) -> (-32.471, 291.6623)
  arc A316 (-46.971, 285.1623) -> (-46.471, 284.6623) centre (-46.471, 285.1623) ccw
  arc A317 (-46.471, 291.6623) -> (-46.971, 291.1623) centre (-46.471, 291.1623) ccw
  arc A318 (-32.471, 284.6623) -> (-31.971, 285.1623) centre (-32.471, 285.1623) ccw
  arc A319 (-31.971, 291.1623) -> (-32.471, 291.6623) centre (-32.471, 291.1623) ccw
  line L324 (-47.971, 329.2555) -> (-47.971, 342.2555)
  line L325 (-33.971, 329.2555) -> (-33.971, 342.2555)
  line L326 (-47.471, 328.7555) -> (-34.471, 328.7555)
  line L327 (-47.471, 342.7555) -> (-34.471, 342.7555)
  arc A320 (-47.971, 329.2555) -> (-47.471, 328.7555) centre (-47.471, 329.2555) ccw
  arc A321 (-47.471, 342.7555) -> (-47.971, 342.2555) centre (-47.471, 342.2555) ccw
  arc A322 (-34.471, 328.7555) -> (-33.971, 329.2555) centre (-34.471, 329.2555) ccw
  arc A323 (-33.971, 342.2555) -> (-34.471, 342.7555) centre (-34.471, 342.2555) ccw
  line L328 (-28.921, 22.0743) -> (-28.921, 35.0743)
  line L329 (-14.921, 22.0742) -> (-14.921, 35.0743)
  line L330 (-28.421, 21.5743) -> (-15.421, 21.5743)
  line L331 (-28.421, 35.5743) -> (-15.421, 35.5743)
  arc A324 (-28.921, 22.0743) -> (-28.421, 21.5742) centre (-28.421, 22.0742) ccw
  arc A325 (-28.421, 35.5743) -> (-28.921, 35.0743) centre (-28.421, 35.0743) ccw
  arc A326 (-15.421, 21.5742) -> (-14.921, 22.0742) centre (-15.421, 22.0742) ccw
  arc A327 (-14.921, 35.0743) -> (-15.421, 35.5743) centre (-15.421, 35.0743) ccw
  line L332 (-28.921, 45.8868) -> (-28.921, 58.8868)
  line L333 (-14.921, 45.8867) -> (-14.921, 58.8868)
  line L334 (-28.421, 45.3868) -> (-15.421, 45.3868)
  line L335 (-28.421, 59.3868) -> (-15.421, 59.3868)
  arc A328 (-28.921, 45.8868) -> (-28.421, 45.3868) centre (-28.421, 45.8868) ccw
  arc A329 (-28.421, 59.3868) -> (-28.921, 58.8868) centre (-28.421, 58.8868) ccw
  arc A330 (-15.421, 45.3868) -> (-14.921, 45.8867) centre (-15.421, 45.8868) ccw
  arc A331 (-14.921, 58.8868) -> (-15.421, 59.3868) centre (-15.421, 58.8868) ccw
  line L336 (-28.921, 69.6993) -> (-28.921, 82.6993)
  line L337 (-14.921, 69.6993) -> (-14.921, 82.6993)
  line L338 (-28.421, 69.1993) -> (-15.421, 69.1993)
  line L339 (-28.421, 83.1993) -> (-15.421, 83.1993)
  arc A332 (-28.921, 69.6993) -> (-28.421, 69.1993) centre (-28.421, 69.6992) ccw
  arc A333 (-28.421, 83.1993) -> (-28.921, 82.6993) centre (-28.421, 82.6993) ccw
  arc A334 (-15.421, 69.1992) -> (-14.921, 69.6993) centre (-15.421, 69.6993) ccw
  arc A335 (-14.921, 82.6993) -> (-15.421, 83.1993) centre (-15.421, 82.6993) ccw
  line L340 (-28.921, 141.1368) -> (-28.921, 154.1368)
  line L341 (-14.921, 141.1368) -> (-14.921, 154.1368)
  line L342 (-28.421, 140.6368) -> (-15.421, 140.6368)
  line L343 (-28.421, 154.6367) -> (-15.421, 154.6368)
  arc A336 (-28.921, 141.1368) -> (-28.421, 140.6368) centre (-28.421, 141.1368) ccw
  arc A337 (-28.421, 154.6367) -> (-28.921, 154.1368) centre (-28.421, 154.1367) ccw
  arc A338 (-15.421, 140.6367) -> (-14.921, 141.1368) centre (-15.421, 141.1368) ccw
  arc A339 (-14.921, 154.1368) -> (-15.421, 154.6368) centre (-15.421, 154.1368) ccw
  line L344 (-27.921, 94.6368) -> (-27.921, 100.6368)
  line L345 (-12.921, 94.6368) -> (-12.921, 100.6368)
  line L346 (-27.421, 94.1368) -> (-13.421, 94.1368)
  line L347 (-27.421, 101.1368) -> (-13.421, 101.1368)
  arc A340 (-27.921, 94.6368) -> (-27.421, 94.1367) centre (-27.421, 94.6368) ccw
  arc A341 (-27.421, 101.1368) -> (-27.921, 100.6368) centre (-27.421, 100.6368) ccw
  arc A342 (-13.421, 94.1368) -> (-12.921, 94.6368) centre (-13.421, 94.6368) ccw
  arc A343 (-12.921, 100.6368) -> (-13.421, 101.1368) centre (-13.421, 100.6368) ccw
  line L348 (-27.921, 194.6368) -> (-27.921, 200.6368)
  line L349 (-12.921, 194.6368) -> (-12.921, 200.6367)
  line L350 (-27.421, 194.1367) -> (-13.421, 194.1368)
  line L351 (-27.421, 201.1368) -> (-13.421, 201.1368)
  arc A344 (-27.921, 194.6368) -> (-27.421, 194.1367) centre (-27.421, 194.6368) ccw
  arc A345 (-27.421, 201.1368) -> (-27.921, 200.6368) centre (-27.421, 200.6368) ccw
  arc A346 (-13.421, 194.1367) -> (-12.921, 194.6368) centre (-13.421, 194.6367) ccw
  arc A347 (-12.921, 200.6368) -> (-13.421, 201.1368) centre (-13.421, 200.6368) ccw
  line L352 (-28.921, 212.5743) -> (-28.921, 225.5743)
  line L353 (-14.921, 212.5743) -> (-14.921, 225.5743)
  line L354 (-28.421, 212.0743) -> (-15.421, 212.0743)
  line L355 (-28.421, 226.0743) -> (-15.421, 226.0742)
  arc A348 (-28.921, 212.5743) -> (-28.421, 212.0743) centre (-28.421, 212.5743) ccw